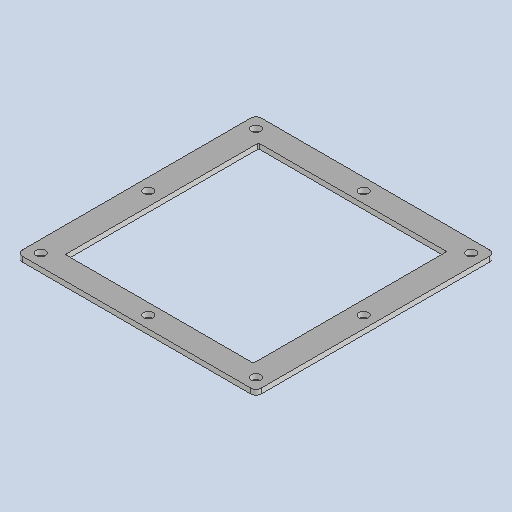
# Autodesk Inventor part: NDV-2103 Collector flange 01
Saved by Autodesk Inventor 2026.2 (Build 302298000, 298)
## iProperties
Created: 2025-06-24
Part Number: NDV-2103 Collector flange 01
Material: Stainless Steel
Document SubType Name: Sheet Metal
Designer: admin
Mass: 62.1684 g
Surface Area: 64.55 cm^2
Volume: 7.77105 cm^3
Density: 8 g/cm^3
Flat Pattern Width: 14 cm
Flat Pattern Length: 14 cm
Flat Pattern Area: 196 cm^2
Sheet Metal Rule: AISI304 2mm Die16
Sheet Metal Width: 140,000 mm
Sheet Metal Length: 140,000 mm
Sheet Metal Area: 19600,000 mm^2
Appearance: Default
Stock Number: Фланец коллектора
Author: user
Autodesk Inventor part; units mm, degrees
ref_plane "YZ Plane" through (0, 0, 0) normal (1, 0, 0) x (0, 1, 0)
ref_plane "XZ Plane" through (0, 0, 0) normal (0, 1, 0) x (-1, 0, 0)
ref_plane "XY Plane" through (0, 0, 0) normal (0, 0, 1) x (1, 0, 0)
sketch "Sketch1" plane through (0, 0, 0) normal (0, 0, 1) x (1, 0, 0)
  line L0 (-70, -70) -> (70, -70)
  line L1 (70, -70) -> (70, 70)
  line L2 (70, 70) -> (-70, 70)
  line L3 (-70, 70) -> (-70, -70)
  line L4 (-70, -70) -> (70, 70) construction
  line L5 (70, -70) -> (-70, 70) construction
  line L6 (55.1, -56.6) -> (-55.1, -56.6)
  line L7 (-55.1, -56.6) -> (-55.1, 56.6)
  line L8 (-55.1, 56.6) -> (55.1, 56.6)
  line L9 (55.1, 56.6) -> (55.1, -56.6)
  line L10 (55.1, -56.6) -> (-55.1, 56.6) construction
  line L11 (-55.1, -56.6) -> (55.1, 56.6) construction
  circle A0 centre (-63, -63) radius 2.75
  circle A1 centre (63, -63) radius 2.75
  circle A2 centre (63, 63) radius 2.75
  circle A3 centre (-63, 63) radius 2.75
  line L12 (65.75, 65.75) -> (-65.75, 65.75) construction
  line L13 (-65.75, 65.75) -> (-65.75, -65.75) construction
  line L14 (-65.75, -65.75) -> (65.75, -65.75) construction
  line L15 (65.75, -65.75) -> (65.75, 65.75) construction
  line L16 (65.75, 65.75) -> (-65.75, -65.75) construction
  line L17 (-65.75, 65.75) -> (65.75, -65.75) construction
  line L18 (63, 63) -> (-63, 63) construction
  line L19 (-63, 63) -> (-63, -63) construction
  line L20 (-63, -63) -> (63, -63) construction
  line L21 (63, -63) -> (63, 63) construction
  line L22 (63, 63) -> (-63, -63) construction
  line L23 (-63, 63) -> (63, -63) construction
  circle A4 centre (0, 63) radius 2.75
  circle A5 centre (-63, 0) radius 2.75
  circle A6 centre (0, -63) radius 2.75
  circle A7 centre (63, 0) radius 2.75
  point P0 (0, 0)
  dimension "d172" = 110.2
  dimension "d190" = 5.5
  dimension "d191" = 126
  dimension "d192" = 140
  dimension "d195" = 113.2
  measures "d172" distance of L7.end L8.end
  measures "d190" diameter of A0
  measures "d191" distance of L19.end L20.end
  measures "d192" distance of L2.end L0.start
  measures "d195" distance of L6.end L7.end
extrude "Plate5" add sketch "Sketch1" along normal blind 3
fillet "Corner Round1" radius 3 4 edges at (70, 70, 1.5) (-70, 70, 1.5) (-70, -70, 1.5) (70, -70, 1.5)
fillet "Corner Round2" radius 0.5 4 edges at (-55.1, 56.6, 1.5) (-55.1, -56.6, 1.5) (55.1, -56.6, 1.5) (55.1, 56.6, 1.5)
derived "NDV-0010 Parameters 01.ipt"
body "Solid3"
